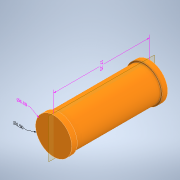
# Autodesk Inventor part: telescopeTube
Saved by Autodesk Inventor 2021 (Build 250183000, 183)
## iProperties
Created: 2020-05-22
Part Number: telescopeTube
Material: Nylon, molybdenum disulphide
Document SubType Name: Modeling
Designer: robst
Density: 1.13 g/cm^3
Appearance: Orange
Author: robst
Autodesk Inventor part; units mm, degrees
ref_plane "XZ Plane" through (0, 0, 0) normal (0, 1, 0) x (-1, 0, 0)
ref_plane "XY Plane" through (0, 0, 0) normal (0, 0, 1) x (1, 0, 0)
sketch "Sketch1" plane through (0, 0, 0) normal (0, 0, 1) x (1, 0, 0)
  circle A0 centre (0, 0) radius 76.2
  dimension "tubeDiameter" = 152.4
  constraints: 1 centre point, 1 coincident
  measures "tubeDiameter" diameter of A0
extrude "Extrusion1" add sketch "Sketch1" along normal mid plane 438.15
sketch "Sketch2" plane through (0, 0, -219.075) normal (0, 0, -1) x (-1, 0, 0)
  circle A0 centre (0, 0) radius 69.85
  dimension "d6" = 139.7
  constraints: 1 centre point, 1 coincident
  measures "d6" diameter of A0
extrude "Extrusion2" cut sketch "Sketch2" against normal blind 406.4
sketch "Sketch3" plane through (0, 0, 219.075) normal (0, 0, 1) x (1, 0, 0)
  circle A0 centre (0, 0) radius 82.55
  circle A1 centre (0, 0) radius 76.2
  dimension "d9" = 165.1
  constraints: 2 centre point, 2 coincident
  measures "d9" diameter of A0
extrude "Extrusion3" add sketch "Sketch3" against normal blind 25.4
sketch "Sketch4" plane through (0, 0, -219.075) normal (0, 0, -1) x (-1, 0, 0)
  circle A0 centre (0, 0) radius 76.2
  circle A1 centre (0, 0) radius 82.55
  constraints: 2 centre point, 2 coincident
extrude "Extrusion4" add sketch "Sketch4" against normal blind 25.4
body "Solid1"
